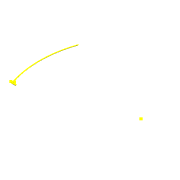
# Autodesk Inventor part: Test_feather_frame
Saved by Autodesk Inventor 2022 (Build 260153000, 153)
## iProperties
Created: 2022-08-06
Part Number: Test_feather_frame
Material: Generic
Document SubType Name: Modeling
Designer: dell
Density: 1 g/cm^3
Appearance: Default
Author: dell
Autodesk Inventor part; units mm, degrees
ref_plane "YZ Plane" through (0, 0, 0) normal (1, 0, 0) x (0, 1, 0)
ref_plane "XZ Plane" through (0, 0, 0) normal (0, 1, 0) x (-1, 0, 0)
ref_plane "XY Plane" through (0, 0, 0) normal (0, 0, 1) x (1, 0, 0)
sketch "Sketch1" plane through (0, 0, 0) normal (0, 1, 0) x (-1, 0, 0)
  line L0 (0, -289.1926) -> (0, 54.5154) projected
  arc A0 (0, -240) -> (0, 0) centre (-350, -120) ccw
  line L1 (0, 0) -> (0, -240)
  line L2 (0, -240) -> (20, -240)
  line L3 (20, -240) -> (20, 0)
  line L4 (20, 0) -> (0, 0)
  arc A1 (1, -240) -> (2, 0) centre (-350.0455, -118.5352) ccw
  line L5 (2, 0) -> (2, 3)
  line L6 (2, 3) -> (-13, 3)
  line L7 (-13, 3) -> (-13, 0)
  line L8 (-13, 0) -> (2, 0)
  point P0 (0, 0)
  dimension "d2" = 240
  dimension "d5" = 20
  dimension "d6" = 2
  dimension "d7" = 1
  dimension "d10" = 3
  dimension "d11" = 15
  constraints: 16 end point, 4 parallel, 4 point on circle, 3 perpendicular, 3 point on line, 2 centre point, 2 tangent, 1 collinear
  measures "d2" distance of L1.start L1.end
  measures "d5" distance between parallel lines of L0 L3
  measures "d6" distance of L1.start L5.start
  measures "d7" distance of L1.end A1.start
  measures "d10" distance between parallel lines of L4 L6
  measures "d11" distance between parallel lines of L5 L7
extrude "Extrusion1" add sketch "Sketch1" along normal blind 2 contours A0 L3 A1 L2 | L8 L7 L6 L0 | L4 A1 L3 A0 | L0 L6 L5 L4 | L3 A1
fillet "Fillet1" radius 4 3 edges at (-2, 1, 3) (-2, 1, 0) (0, 1, 0)
sketch "Sketch2" plane through (0, 2, 0) normal (0, 1, 0) x (1, 0, 0)
  line L0 (13, 0) -> (2.8689, 0) projected
  arc A0 (0, 240) -> (-0.9249, 2.7322) centre (350, 120) ccw projected
  line L1 (0, 240) -> (-1, 240) projected
  arc A1 (-1, 240) -> (-2.2069, 0.6162) centre (350.0455, 118.5352) ccw projected
  line L2 (1.8272, -3) -> (13, -3) projected
  line L3 (13, -3) -> (13, 0) projected
  arc A2 (-2.0864, 0.1732) -> (1.8272, -3) centre (1.8272, 1) ccw projected
  arc A3 (-2.0864, 0.1732) -> (-2.2069, 0.6162) centre (-6, -0.6535) ccw projected
  arc A4 (-0.9249, 2.7322) -> (2.8689, 0) centre (2.8689, 4) ccw projected
  point P0 (0, 0)
body "Solid1"
